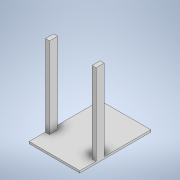
# Autodesk Inventor part: Catapult
Saved by Autodesk Inventor 2022.2 (Build 262287000, 287)
## iProperties
Created: 2022-01-16
Part Number: Catapult
Material: Generic
Document SubType Name: Modeling
Designer: robst
Density: 1 g/cm^3
Appearance: Default
Author: robst
Autodesk Inventor part; units mm, degrees
ref_plane "YZ Plane" through (0, 0, 0) normal (1, 0, 0) x (0, 1, 0)
ref_plane "XZ Plane" through (0, 0, 0) normal (0, 1, 0) x (-1, 0, 0)
ref_plane "XY Plane" through (0, 0, 0) normal (0, 0, 1) x (1, 0, 0)
sketch "Sketch1" plane through (0, 0, 0) normal (0, 1, 0) x (-1, 0, 0)
  line L0 (317.5, 444.5) -> (-317.5, 444.5)
  line L1 (-317.5, 444.5) -> (-317.5, -444.5)
  line L2 (-317.5, -444.5) -> (317.5, -444.5)
  line L3 (317.5, -444.5) -> (317.5, 444.5)
  line L4 (317.5, 444.5) -> (-317.5, -444.5) construction
  line L5 (-317.5, 444.5) -> (317.5, -444.5) construction
  point P0 (0, 0)
  dimension "d0" = 635
  dimension "d1" = 889
  constraints: 12 end point, 2 midpoint, 2 parallel, 1 horizontal, 1 perpendicular
  measures "d0" distance of L0.start L0.end
  measures "d1" distance of L1.end L0.end
extrude "Extrusion1" add sketch "Sketch1" against normal blind 25.4
sketch "Sketch2" plane through (0, 0, 0) normal (0, 1, 0) x (1, 0, 0)
  line L0 (-317.5, -444.5) -> (-317.5, 444.5) projected
  line L1 (-317.5, -241.3) -> (-266.7, -241.3)
  line L2 (-266.7, -241.3) -> (-266.7, -139.7)
  line L3 (-266.7, -139.7) -> (-317.5, -139.7)
  line L4 (-317.5, -139.7) -> (-317.5, -241.3)
  line L5 (-317.5, -444.5) -> (317.5, -444.5) projected
  point P0 (0, 0)
  dimension "d6" = 101.6
  dimension "d7" = 50.8
  dimension "d8" = 203.2
  constraints: 8 end point, 2 parallel, 1 horizontal, 1 perpendicular, 1 point on line
  measures "d6" distance of L1.end L2.end
  measures "d7" distance of L1.start L1.end
  measures "d8" distance between parallel lines of L1 L5
extrude "Extrusion2" add sketch "Sketch2" along normal blind 1016
mirror "Mirror1" about plane through (0, 0, 0) normal (1, 0, 0) of "Extrusion2"
body "Solid1"
